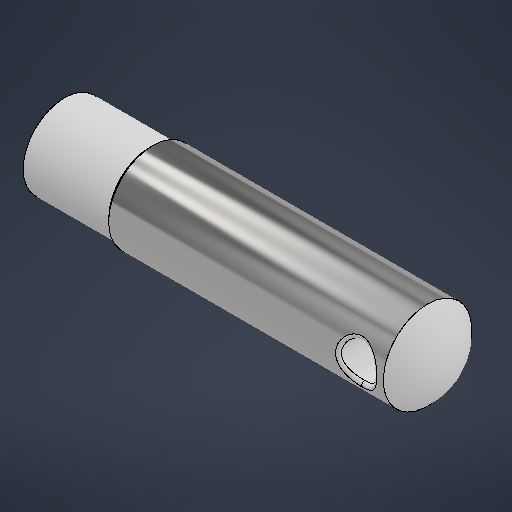
# Autodesk Inventor part: TW2A-004A
Saved by Autodesk Inventor 2025.3 (Build 293356000, 356)
## iProperties
Created: 2025-05-04
Part Number: TW2A-004A
Material: Generic
Document SubType Name: Modeling
Designer: fablabadmin
Density: 1 g/cm^3
Appearance: Default
Description: Handle
Stock Number: C45E
Author: Benjamin Solar
Title: WEDU
Revision Number: 1
Autodesk Inventor part; units mm, degrees
ref_plane "YZ Plane" through (0, 0, 0) normal (1, 0, 0) x (0, 1, 0)
ref_plane "XZ Plane" through (0, 0, 0) normal (0, 1, 0) x (-1, 0, 0)
ref_plane "XY Plane" through (0, 0, 0) normal (0, 0, 1) x (1, 0, 0)
sketch "Sketch1" plane through (0, 0, 0) normal (0, 0, 1) x (1, 0, 0)
  line L0 (-13.1614, 0) -> (78.9686, 0) projected
  line L1 (0, -5.1729) -> (0, 10.0373) projected
  line L2 (0, 7) -> (15, 7)
  line L3 (15, 7) -> (15, 7.5)
  line L4 (15, 7.5) -> (61.6144, 7.5)
  line L5 (61.6144, 7.5) -> (61.6144, 0) construction
  line L6 (0, 5.1) -> (47.0555, 5.1)
  line L7 (47.0555, 5.1) -> (50, 0)
  arc A0 (65, 0) -> (61.6144, 7.5) centre (55, 0) ccw
  circle A1 centre (57, 0) radius 3
  line L8 (15, 7.5) -> (14.5, 7)
  point P0 (0, 0)
  dimension "d0" = 10.2
  dimension "d3" = 15
  dimension "d6" = 50
  dimension "d8" = 15
  dimension "d9" = 10
  dimension "d10" = 6
  dimension "d12" = 65
  dimension "d13" = 0.5
  dimension "d14" = 0.5
  dimension "d15" = 57
  dimension "d19" = 14
  dimension "d20" = 60
  dimension "d21" = 3.3856
  constraints: 14 end point, 8 point on line, 3 perpendicular, 2 centre point, 2 horizontal, 2 point on circle
  measures "d0" diameter of L6 L0
  measures "d3" diameter of L4 L0
  measures "d6" distance from line of L1 L7.end
  measures "d8" distance of L2.start L2.end
  measures "d9" radius of A0
  measures "d10" diameter of A1
  measures "d12" distance from line of A0.start L1
  measures "d13" horizontal distance of L8.end L3.end
  measures "d14" distance of L2.end L3.end
  measures "d15" distance from line of A1.centre L1
  measures "d19" diameter of L2 L0
  measures "d20" angle of L7 L0
  measures "d21" distance of L5.end A0.start
revolve "Revolution1" add sketch "Sketch1" angle 360 about axis through (-10, 0, 0) along (1, 0, 0) picked at (56.166, 1.3672) contours A1 L0 L7 L6 L1 L2 L3 L4 A0 | L0 A1 | L3 L2 L8
extrude "Extrusion1" cut sketch "Sketch1" along normal through all both and the other way through all contours A1 L0 | L0 A1
fillet "Fillet1" radius 0.5 2 edges at (54, 0.0092, 7.5) (54, 0.0092, -7.5)
equation "\"d13\" = d14"
body "Solid1"
